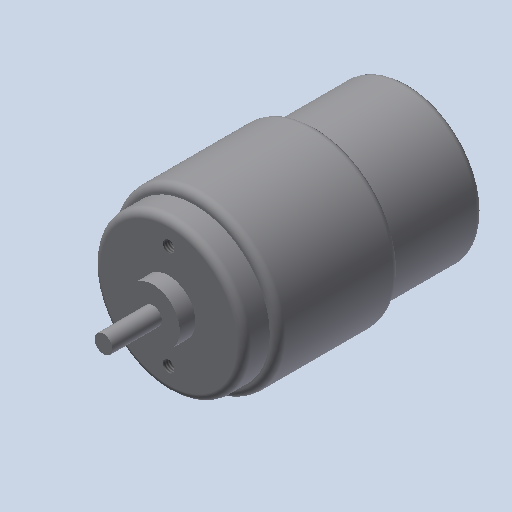
# Autodesk Inventor part: 775
Saved by Autodesk Inventor 2022 (Build 260153000, 153)
## iProperties
Shininess: 64.0
Length Units: 11269
Angle Units: 11279
Time Units: 11290
Mass Units: 11284
Length Display Precision: 3
Angle Display Precision: 2
Compacted: True
Part Number: 775
Document SubType Name: Modeling
Created: 2007-10-30
Designer: takahiro
Manufacturer: Standard
Standards Organization: Custom
Material: 一般
Density: 1 g/cm^3
Appearance: 既定
Density: 0.0
Volumn: 0.0
Area: 0.0
PropertySet Name: Model Information
Control State: 0
Master: False
Checked Out: False
Author: takahiro
Autodesk Inventor part; units mm, degrees
ref_plane "YZ Plane" through (0, 0, 0) normal (1, 0, 0) x (0, 1, 0)
ref_plane "XZ Plane" through (0, 0, 0) normal (0, 1, 0) x (-1, 0, 0)
sketch "スケッチ1" plane through (0, 0, 0) normal (0, 0, 1) x (1, 0, 0)
  circle A0 centre (0, 0) radius 2.5
  dimension "d0" = 5
  constraints: 1 centre point
  measures "d0" diameter of A0
extrude "押し出し1" add sketch "スケッチ1" along normal blind 18.2
sketch "スケッチ2" plane through (0, 0, 0) normal (0, 0, -1) x (-1, 0, 0)
  circle A0 centre (0, 0) radius 2.5 projected
  circle A1 centre (0, 0) radius 7.5
  dimension "d3" = 15
  constraints: 1 centre point, 1 coincident
  measures "d3" diameter of A1
extrude "押し出し2" add sketch "スケッチ2" against normal blind 4.4
sketch "スケッチ3" plane through (0, 0, 0) normal (0, 0, -1) x (-1, 0, 0)
  circle A0 centre (0, 0) radius 7.5 projected
  circle A1 centre (0, 0) radius 21.05
  dimension "d6" = 42.1
  constraints: 1 centre point, 1 coincident
  measures "d6" diameter of A1
extrude "押し出し3" add sketch "スケッチ3" along normal blind 67 contours A0 | A1
ref_plane "作業平面1" through (0, 0, -7.2) normal (0, 0, 1) x (1, 0, 0)
sketch "スケッチ6" plane through (0, 0, -7.2) normal (0, 0, 1) x (1, 0, 0)
  circle A0 centre (0, 0) radius 23.5
  dimension "d14" = 47
  constraints: 1 centre point
  measures "d14" diameter of A0
extrude "押し出し5" add sketch "スケッチ6" against normal blind 34
sketch "スケッチ7" plane through (0, 0, 0) normal (0, 0, 1) x (1, 0, 0)
  circle A0 centre (0, 14.5) radius 0.9915
  circle A1 centre (0, 0) radius 2.5 projected
  dimension "d17" = 14.5
  constraints: 1 centre point
  measures "d17" distance of A1.centre A0.centre
hole "穴1" at (0, 14.5, 0) direction (0, 0, -1) diameter 3.242 depth 8 tip angle 118 thread size "M4x0.7" class "6H" standard "ISO Metric profile"
pattern_circular "放射状パターン1" count 2 over 360 about axis through (0, 0, 0) along (0, 0, 1) of "穴1"
fillet "フィレット1" radius 2 1 edges at (21.05, 0, 0)
fillet "フィレット2" radius 2 2 edges at (-23.5, 0, -7.2) (-23.5, 0, -41.2)
fillet "フィレット3" radius 2 1 edges at (21.05, 0, -67)
